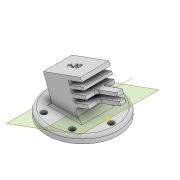
# Autodesk Inventor part: Plate_20
Saved by Autodesk Inventor 2022 (Build 260153000, 153)
## iProperties
Created: 2022-12-25
Part Number: Plate_20
Material: Generic
Document SubType Name: Modeling
Designer: dell
Density: 1 g/cm^3
Appearance: Default
Author: dell
Autodesk Inventor part; units mm, degrees
ref_plane "YZ Plane" through (0, 0, 0) normal (1, 0, 0) x (0, 1, 0)
ref_plane "XZ Plane" through (0, 0, 0) normal (0, 1, 0) x (-1, 0, 0)
ref_plane "XY Plane" through (0, 0, 0) normal (0, 0, 1) x (1, 0, 0)
sketch "Sketch1" plane through (0, 0, 0) normal (0, 1, 0) x (-1, 0, 0)
  circle A0 centre (0, 0) radius 50
  dimension "d0" = 100
  constraints: 1 centre point, 1 coincident
  measures "d0" diameter of A0
extrude "Extrusion1" add sketch "Sketch1" along normal blind 10
sketch "Sketch2" plane through (0, 10, 0) normal (0, 1, 0) x (1, 0, 0)
  circle A0 centre (-40, 0) radius 4.1
  point P0 (0, 0)
  dimension "d3" = 8.2
  dimension "d4" = 40
  constraints: 1 centre point
  measures "d3" diameter of A0
  measures "d4" distance of point (0, 0) A0.centre
extrude "Extrusion2" cut sketch "Sketch2" against normal blind 100
pattern_circular "Circular Pattern1" count 6 over 360 about axis through (0, 0, 0) along (0, 1, 0) of "Extrusion2"
ref_plane "Work Plane1" through (0, 10, -10) normal (0.3420201, -0.9396926, 0) x (0, 0, 1)
sketch "Sketch3" plane through (0, 10, 0) normal (-0.3420201, 0.9396926, 0) x (0.9396926, 0.3420201, 0)
  line L0 (-20.9202, 20) -> (14.0798, 20)
  line L1 (14.0798, 20) -> (14.0798, -20)
  line L2 (14.0798, -20) -> (-20.9202, -20)
  line L3 (-20.9202, -20) -> (-20.9202, 20)
  line L4 (-20.9202, 20) -> (14.0798, -20) construction
  line L5 (14.0798, 20) -> (-20.9202, -20) construction
  point P0 (-3.4202, 0)
  dimension "d10" = 35
  dimension "d11" = 40
  constraints: 12 end point, 2 midpoint, 2 parallel, 1 horizontal, 1 perpendicular
  measures "d10" distance of L1.end L2.end
  measures "d11" distance of L0.end L1.end
extrude "Extrusion3" add sketch "Sketch3" along normal blind 45
sketch "Sketch5" plane through (14.9834, 10, 20) normal (0.9396926, 0.3420201, 0) x (0, 0, -1)
  line L0 (0, 5.1246) -> (0, 50.1246) projected
  line L1 (40, 12.739) -> (40, 50.1246) projected
  line L2 (0, 20.1246) -> (40, 20.1246)
  line L3 (40, 20.1246) -> (40, 15.1246)
  line L4 (40, 15.1246) -> (0, 15.1246)
  line L5 (0, 15.1246) -> (0, 20.1246)
  line L6 (0, 12.739) -> (0, 50.1246) projected
  line L7 (0, 25.1246) -> (40, 25.1246)
  line L8 (40, 25.1246) -> (40, 30.1246)
  line L9 (40, 30.1246) -> (0, 30.1246)
  line L10 (0, 30.1246) -> (0, 25.1246)
  line L11 (40, 12.739) -> (40, 50.1246) projected
  line L12 (0, 39.3246) -> (40, 39.3246)
  line L13 (40, 39.3246) -> (40, 35.1246)
  line L14 (40, 35.1246) -> (0, 35.1246)
  line L15 (0, 35.1246) -> (0, 39.3246)
  line L16 (0, 44.3246) -> (40, 44.3246)
  line L17 (40, 5.1246) -> (40, 50.1246) projected
  line L18 (0, 50.1246) -> (40, 50.1246) projected
  line L19 (0, 5.1246) -> (0, 50.1246) projected
  line L20 (0, 5.1246) -> (40, 5.1246) projected
  point P0 (20, -4.2723)
  point P1 (0, 0)
  point P2 (0, 15.1246)
  point P3 (40, 20.1246)
  point P4 (0, 44.3246)
  point P5 (0, 35.1246)
  point P6 (40, 39.3246)
  point P7 (0, 39.3246)
  point P8 (0, 30.1246)
  point P9 (0, 25.1246)
  dimension "d16" = 5
  dimension "d19" = 5
  dimension "d20" = 5
  dimension "d21" = 5
  dimension "d22" = 4.2
  dimension "d23" = 5
  dimension "d44" = 15
  constraints: 26 end point, 8 point on line, 6 parallel, 4 perpendicular, 3 horizontal
  measures "d16" distance between parallel lines of L2 L4
  measures "d19" distance between parallel lines of L7 L2
  measures "d20" distance between parallel lines of L7 L9
  measures "d21" distance between parallel lines of L9 L14
  measures "d22" distance between parallel lines of L14 L12
  measures "d23" distance between parallel lines of L12 L16
  measures "d44" distance between parallel lines of L20 L2
extrude "Extrusion4" add sketch "Sketch5" along normal blind 20 contours L0 L2 L1 L4 | L0 L9 L1 L7 | L0 L12 L1 L14 | L0 L18 L1 L16
sketch "Sketch7" plane through (33.7773, 16.8404, 20) normal (0.9396926, 0.3420201, 0) x (0, 0, -1)
  point P0 (20, -4.2723)
sketch "Sketch6" plane through (33.7773, 16.8404, 20) normal (0.9396926, 0.3420201, 0) x (0, 0, -1)
  line L0 (40, 15.1246) -> (40, 20.1246) projected
  line L1 (40, 20.1246) -> (0, 20.1246) projected
  line L2 (0, 20.1246) -> (0, 15.1246) projected
  line L3 (0, 15.1246) -> (40, 15.1246) projected
  line L4 (0, 30.1246) -> (0, 25.1246) projected
  line L5 (0, 25.1246) -> (40, 25.1246) projected
  line L6 (40, 25.1246) -> (40, 30.1246) projected
  line L7 (40, 30.1246) -> (0, 30.1246) projected
  line L8 (40, 30.1246) -> (0, 30.1246) projected
  line L9 (15.4, 30.1246) -> (24.6, 30.1246)
  line L10 (24.6, 30.1246) -> (24.6, 25.1246)
  line L11 (24.6, 25.1246) -> (15.4, 25.1246)
  line L12 (15.4, 25.1246) -> (15.4, 30.1246)
  line L13 (40, 20.1246) -> (0, 20.1246) projected
  line L14 (15.4, 20.1246) -> (24.6, 20.1246)
  line L15 (24.6, 20.1246) -> (24.6, 15.1246)
  line L16 (24.6, 15.1246) -> (15.4, 15.1246)
  line L17 (15.4, 15.1246) -> (15.4, 20.1246)
  line L18 (20, -40.2309) -> (20, 91.7723) projected
  point P0 (20, -4.2723)
  point P1 (15.4, 15.1246)
  point P2 (24.6, 30.1246)
  point P3 (15.4, 30.1246)
  dimension "d24" = 9.2
  dimension "d25" = 9.2
  dimension "d26" = 4.6
  dimension "d27" = 4.6
  constraints: 16 end point, 4 parallel, 4 point on line, 2 horizontal, 2 perpendicular
  measures "d24" distance between parallel lines of L10 L12
  measures "d25" distance between parallel lines of L17 L15
  measures "d26" distance between parallel lines of L18 L12
  measures "d27" distance between parallel lines of L18 L17
extrude "Extrusion5" add sketch "Sketch6" along normal blind 30 contours L3 L18 L1 L15 | L3 L17 L1 L18 | L7 L18 L5 L12 | L7 L10 L5 L18
thicken "Thicken1" operation add thickness 0.2 both sides no extend neighbours yes toward (0.3420201, -0.9396926, 0) faces at (14.365, 31.1911, -1.5333)
thicken "Thicken2" operation add thickness 0.2 both sides no extend neighbours yes toward (-0.3420201, 0.9396926, 0) faces at (12.6549, 35.8896, -1.5333)
thicken "Thicken3" operation add thickness 0.2 both sides no extend neighbours yes toward (0.3420201, -0.9396926, 0) faces at (10.9448, 40.588, -1.5333)
thicken "Thicken4" operation add thickness 0.2 both sides no extend neighbours yes toward (-0.3420201, 0.9396926, 0) faces at (9.2347, 45.2865, 6.6667)
thicken "Thicken5" operation add thickness 0.2 both sides no extend neighbours yes toward (0.3420201, -0.9396926, 0) faces at (7.7982, 49.2332, -6.6667)
thicken "Thicken6" operation add thickness 0.2 both sides no extend neighbours yes toward (-0.3420201, 0.9396926, 0) faces at (6.0881, 53.9317, -6.6667)
fillet "Fillet1" radius 3 8 edges at (-22.2628, 10, 0) (-11.1314, 10, -20) (-11.1314, 10, 20) (9.8105, 24.2125, 0) (27.7835, 33.3082, -4.6) (24.3291, 42.7991, -4.6) (24.3291, 42.7991, 4.6) (27.7835, 33.3082, 4.6)
chamfer "Chamfer1" distance 14 angle 45 3 edges at (0, 10, -21.5) (0, 10, 0) (0, 10, 21.5)
fillet "Fillet3" radius 10 3 edges at (14, 10, 0) (14, 10, 21.5) (14, 10, -21.5)
fillet "Fillet4" radius 4 1 edges at (50, 10, 0)
sketch "Sketch8" plane through (-15.3909, 52.2862, 0) normal (-0.3420201, 0.9396926, 0) x (0.9396926, 0.3420201, 0)
  line L0 (-6.9685, 4.6888) -> (10.8183, 4.6888) construction
  line L1 (10.8183, 4.6888) -> (10.8183, -13.2224) construction
  line L2 (10.8183, -13.2224) -> (-6.9685, -13.2224) construction
  line L3 (-6.9685, -13.2224) -> (-6.9685, 4.6888) construction
  line L4 (0.1952, -0.4069) -> (-2.5147, -0.4069)
  line L5 (-2.5147, -0.4069) -> (-2.5147, -3.1167)
  line L6 (-2.5147, -3.1167) -> (-3.4093, -3.1167)
  line L7 (-3.4093, -3.1167) -> (-3.4093, -0.4069)
  line L8 (-3.4093, -0.4069) -> (-6.1192, -0.4069)
  line L9 (-6.1192, -0.4069) -> (-6.1192, 0.4554)
  line L10 (-6.1192, 0.4554) -> (-3.4093, 0.4554)
  line L11 (-3.4093, 0.4554) -> (-3.4093, 3.1653)
  line L12 (-3.4093, 3.1653) -> (-2.5147, 3.1653)
  line L13 (-2.5147, 3.1653) -> (-2.5147, 0.4554)
  line L14 (-2.5147, 0.4554) -> (0.1952, 0.4554)
  line L15 (0.1952, 0.4554) -> (0.1952, -0.4069)
  line L16 (6.555, -3.4798) -> (1.6215, -3.4798)
  line L17 (1.6215, -3.4798) -> (1.6215, -2.3453)
  spline S0 degree 2 poles (1.6215, -2.3453) (2.1531, -1.8461) (3.0996, -0.919) (3.5534, -0.4198) knots 0 0 0 1 2 2 2
  spline S1 degree 2 poles (3.5534, -0.4198) (4.4675, 0.585) (5.1352, 1.7909) (5.1352, 2.4327) knots 0 0 0 1 2 2 2
  spline S2 degree 2 poles (5.1352, 2.4327) (5.1352, 2.7698) (4.9278, 3.2755) (4.7398, 3.4375) knots 0 0 0 1 2 2 2
  spline S3 degree 2 poles (4.7398, 3.4375) (4.5518, 3.5996) (4.0591, 3.7617) (3.7608, 3.7617) knots 0 0 0 1 2 2 2
  spline S4 degree 2 poles (3.7608, 3.7617) (3.4756, 3.7617) (2.8921, 3.6191) (2.6263, 3.5089) knots 0 0 0 1 2 2 2
  spline S5 degree 2 poles (2.6263, 3.5089) (2.3994, 3.4181) (1.978, 3.1588) (1.8484, 3.068) knots 0 0 0 1 2 2 2
  line L18 (1.8484, 3.068) -> (1.79, 3.068)
  line L19 (1.79, 3.068) -> (1.79, 4.209)
  spline S6 degree 2 poles (1.79, 4.209) (2.1206, 4.3711) (3.307, 4.6888) (3.8386, 4.6888) knots 0 0 0 1 2 2 2
  spline S7 degree 2 poles (3.8386, 4.6888) (4.9602, 4.6888) (6.2244, 3.5024) (6.2244, 2.491) knots 0 0 0 1 2 2 2
  spline S8 degree 2 poles (6.2244, 2.491) (6.2244, 2.0178) (6.0039, 1.2269) (5.8095, 0.8897) knots 0 0 0 1 2 2 2
  spline S9 degree 2 poles (5.8095, 0.8897) (5.615, 0.5397) (5.0509, -0.1475) (4.7398, -0.4782) knots 0 0 0 1 2 2 2
  spline S10 degree 2 poles (4.7398, -0.4782) (4.2341, -1.0292) (2.9958, -2.2091) (2.6263, -2.5527) knots 0 0 0 1 2 2 2
  line L20 (2.6263, -2.5527) -> (6.555, -2.5527)
  line L21 (6.555, -2.5527) -> (6.555, -3.4798)
  spline S11 degree 2 poles (12.6036, 0.5202) (12.6036, -1.6321) (11.3524, -3.6484) (10.0493, -3.6484) knots 0 0 0 1 2 2 2
  spline S12 degree 2 poles (10.0493, -3.6484) (8.7268, -3.6484) (7.4886, -1.5932) (7.4886, 0.5137) knots 0 0 0 1 2 2 2
  spline S13 degree 2 poles (7.4886, 0.5137) (7.4886, 2.679) (8.7398, 4.6823) (10.0493, 4.6823) knots 0 0 0 1 2 2 2
  spline S14 degree 2 poles (10.0493, 4.6823) (11.3654, 4.6823) (12.6036, 2.6077) (12.6036, 0.5202) knots 0 0 0 1 2 2 2
  spline S15 degree 2 poles (11.2292, -1.9174) (11.3848, -1.5219) (11.5145, -0.3031) (11.5145, 0.5202) knots 0 0 0 1 2 2 2
  spline S16 degree 2 poles (11.5145, 0.5202) (11.5145, 1.3435) (11.3848, 2.5559) (11.2227, 2.9643) knots 0 0 0 1 2 2 2
  spline S17 degree 2 poles (11.2227, 2.9643) (11.0607, 3.3727) (10.4967, 3.7941) (10.0493, 3.7941) knots 0 0 0 1 2 2 2
  spline S18 degree 2 poles (10.0493, 3.7941) (9.602, 3.7941) (9.025, 3.3727) (8.8565, 2.9513) knots 0 0 0 1 2 2 2
  spline S19 degree 2 poles (8.8565, 2.9513) (8.6944, 2.5429) (8.5777, 1.2982) (8.5777, 0.5137) knots 0 0 0 1 2 2 2
  spline S20 degree 2 poles (8.5777, 0.5137) (8.5777, -0.3291) (8.6814, -1.4571) (8.85, -1.8979) knots 0 0 0 1 2 2 2
  spline S21 degree 2 poles (8.85, -1.8979) (9.0056, -2.3129) (9.5826, -2.7602) (10.0493, -2.7602) knots 0 0 0 1 2 2 2
  spline S22 degree 2 poles (10.0493, -2.7602) (10.4902, -2.7602) (11.0672, -2.3388) (11.2292, -1.9174) knots 0 0 0 1 2 2 2
  point P0 (-3.4202, 0)
  constraints: 2 other
extrude "Extrusion6" cut sketch "Sketch8" against normal blind 1
fillet "Fillet5" radius 1 4 edges at (55.9743, 43.5688, 4.6) (52.5199, 53.0597, 4.6) (52.5199, 53.0597, -4.6) (55.9743, 43.5688, -4.6)
equation "\"d26\" = 0.5 * d24"
equation "\"d27\" = 0.5 * d25"
body "Solid1"
